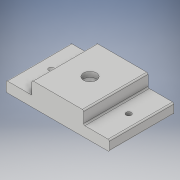
# Autodesk Inventor part: Base
Saved by Autodesk Inventor 2019 (Build 230136000, 136)
## iProperties
Created: 2019-02-14
Part Number: Base
Material: Generic
Document SubType Name: Modeling
Designer: lopez.xavier
Density: 1 g/cm^3
Appearance: Default
Author: lopez.xavier
Autodesk Inventor part; units mm, degrees
ref_plane "YZ Plane" through (0, 0, 0) normal (1, 0, 0) x (0, 1, 0)
ref_plane "XZ Plane" through (0, 0, 0) normal (0, 1, 0) x (-1, 0, 0)
ref_plane "XY Plane" through (0, 0, 0) normal (0, 0, 1) x (1, 0, 0)
sketch "Sketch1" plane through (0, 0, 0) normal (0, 0, 1) x (1, 0, 0)
  line L0 (0, 0) -> (50.8, 0)
  line L1 (50.8, 0) -> (50.8, 5.08)
  line L2 (50.8, 5.08) -> (0, 5.08)
  line L3 (0, 5.08) -> (0, 0)
  line L4 (12.7, 5.08) -> (38.1, 5.08)
  line L5 (38.1, 5.08) -> (38.1, 11.43)
  line L6 (38.1, 11.43) -> (12.7, 11.43)
  line L7 (12.7, 11.43) -> (12.7, 5.08)
  dimension "d0" = 50.8
  dimension "d1" = 5.08
  dimension "d2" = 25.4
  dimension "d3" = 6.35
  dimension "d4" = 12.7
  constraints: 16 end point, 4 parallel, 2 horizontal, 2 perpendicular, 1 point on line
  measures "d0" distance of L2.end L1.end
  measures "d1" distance of L1.end L0.end
  measures "d2" distance of L6.end L5.end
  measures "d3" distance of L5.end L4.end
  measures "d4" distance of L2.end L4.start
extrude "Extrusion1" add sketch "Sketch1" along normal blind 31.75
sketch "Sketch3" plane through (12.7, 11.43, 0) normal (0, 1, 0) x (1, 0, 0)
  circle A0 centre (12.7, -15.875) radius 3.175
  line L0 (25.4, 0) -> (0, 0) projected
  line L1 (25.4, 0) -> (25.4, -31.75) projected
  point P0 (-12.7, 0)
  dimension "d8" = 15.875
  dimension "d9" = 12.7
  dimension "d20" = 6.35
  constraints: 1 centre point
  measures "d8" distance from line of L0 A0.centre
  measures "d9" distance from line of L1 A0.centre
  measures "d20" diameter of A0
extrude "Extrusion2" cut sketch "Sketch3" against normal blind 2.54
sketch "Sketch4" plane through (0, 5.08, 0) normal (0, 1, 0) x (1, 0, 0)
  circle A0 centre (6.35, -15.875) radius 1.27
  circle A1 centre (44.45, -15.875) radius 1.27
  line L0 (50.8, 0) -> (50.8, -31.75) projected
  line L1 (0, 0) -> (0, -31.75) projected
  line L2 (50.8, 0) -> (38.1, 0) projected
  line L3 (12.7, 0) -> (0, 0) projected
  dimension "d12" = 2.54
  dimension "d13" = 2.54
  dimension "d14" = 6.35
  dimension "d15" = 6.35
  dimension "d16" = 15.875
  dimension "d17" = 15.875
  constraints: 2 centre point
  measures "d12" diameter of A0
  measures "d13" diameter of A1
  measures "d14" distance from line of L0 A1.centre
  measures "d15" distance from line of L1 A0.centre
  measures "d16" distance from line of L2 A1.centre
  measures "d17" distance from line of L3 A0.centre
extrude "Extrusion3" cut sketch "Sketch4" against normal blind 25.4
fillet "Fillet1" radius 0.635 8 edges at (12.7, 11.43, 15.875) (38.1, 11.43, 15.875) (38.1, 5.08, 15.875) (50.8, 5.08, 15.875) (0, 5.08, 15.875) (50.8, 0, 15.875) (0, 0, 15.875) (12.7, 5.08, 15.875)
equation "\"d12\" = d13"
equation "\"d15\" = d14"
equation "\"d17\" = d16"
body "Solid1"
